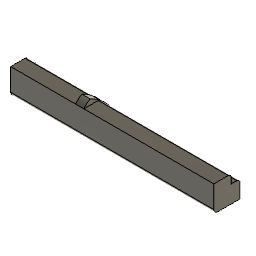
key (Autodesk Fusion 360 design; units mm, degrees)
part number: 2026-04-09-15-21-44-763
Autodesk Fusion 360 part; units mm, degrees
note: some values were not read from the file. Set by a fixed rule: which sketch regions a step uses.
sketch "Sketch1" plane through (0, 0, 0) normal (0, 0, 1) x (1, 0, 0)
  line L0 (0, 0) -> (52, 0)
  line L1 (52, 0) -> (52, 6.7)
  line L2 (52, 6.7) -> (0, 6.7)
  line L3 (0, 6.7) -> (0, 0)
  dimension "d1" = 52
  dimension "d2" = 6.7
  constraint horizontal L0
  constraint vertical L1
  constraint horizontal L2
  constraint vertical L3
  constraint coincident L0.start L3.end
  measures "d1" distance of L0.start L0.end
  measures "d2" distance of L0.start L2.end
extrude "Extrude1" add sketch "Sketch1" along normal blind 6.7
sketch "Sketch2" plane through (0, 0, 6.7) normal (0, 0, 1) x (-1, 0, 0)
  line L0 (0, -6.7) -> (0, 0)
  line L1 (0, 0) -> (-52, 0)
  line L2 (-52, 0) -> (-52, -6.7)
  line L3 (-52, -6.7) -> (0, -6.7)
  line L4 (0, 0) -> (-52, 0)
  line L5 (-52, 0) -> (-52, -4.45)
  line L6 (-52, -4.45) -> (0, -4.45)
  line L7 (0, -4.45) -> (0, 0)
  dimension "d5" = 4.45
  constraint horizontal L4
  constraint vertical L5
  constraint horizontal L6
  constraint vertical L7
  constraint coincident L0.end L1.start
  measures "d5" distance of L0.end L6.end
extrude "Extrude2" cut sketch "Sketch2" against normal blind 2.25 contours L0 L2 L3 L6
fillet "Fillet2" radius 0.75 2 edges at (26, 6.7, 4.45) (26, 4.45, 6.7)
fillet "Fillet3" radius 1 1 edges at (26, 0, 0)
ref_plane "WorkPlane2" through (18.75, 0, 0) normal (1, 0, 0) x (0, 1, 0)
sketch "Sketch8" plane through (18.75, 0, 0) normal (1, 0, 0) x (0, 1, 0)
  line L0 (4.45, 4.45) -> (6.7, 2.2) construction
  line L1 (4.45, 4.45) -> (2.1892, 6.7108) construction
  line L2 (0, 6.7) -> (1.6, 6.7) construction
  line L3 (6.7, 0) -> (6.7, 1.6) construction
  line L4 (6.7, 1.6) -> (8.1, 1.6) construction
  line L5 (1.6, 6.7) -> (1.6, 8.1) construction
  line L6 (4.45, 4.45) -> (7, 7) construction
  line L7 (5.575, 3.325) -> (8.1813, 5.9313) construction
  line L8 (3.3196, 5.5804) -> (5.5098, 7.7707) construction
  arc A0 (6.7, 0) -> (8.1, 1.6) centre (2.6, 5) ccw
  arc A1 (1.6, 8.1) -> (0, 6.7) centre (5, 2.6) ccw
  line L9 (0, 6.7) -> (6.7, 0)
  arc A2 (8.1, 1.6) -> (1.6, 8.1) centre (-4.0249, -4.0249) ccw
  dimension "d18" = 1.6
  dimension "d19" = 1.6
  dimension "d20" = 1.4
  dimension "d21" = 1.4
  constraint parallel L0 L1
  constraint horizontal L2
  constraint vertical L3
  constraint perpendicular L3 L4
  constraint perpendicular L2 L5
  constraint perpendicular L0 L6
  constraint midpoint L0 L7.start
  constraint perpendicular L0 L7
  constraint midpoint L1 L8.start
  constraint perpendicular L1 L8
  measures "d18" distance of L2.start L2.end
  measures "d19" distance of L3.start L3.end
  measures "d20" distance of L3.end L4.end
  measures "d21" distance of L2.end L5.end
extrude "Extrude3" add sketch "Sketch8" against normal blind 2.1
